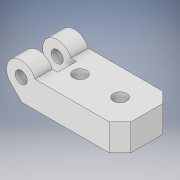
# Autodesk Inventor part: Piston Wall Guide
Saved by Autodesk Inventor 2018 (Build 220112000, 112)
## iProperties
Created: 2017-09-27
Part Number: Piston Wall Guide
Material: ASA Plastic
Document SubType Name: Modeling
Designer: Gabriel Smolnycki
Density: 1.07 g/cm^3
Appearance: Smooth - White ASA
Author: Gabriel Smolnycki
Autodesk Inventor part; units mm, degrees
ref_plane "YZ Plane" through (0, 0, 0) normal (1, 0, 0) x (0, 1, 0)
ref_plane "XZ Plane" through (0, 0, 0) normal (0, 1, 0) x (-1, 0, 0)
ref_plane "XY Plane" through (0, 0, 0) normal (0, 0, 1) x (1, 0, 0)
sketch "Sketch1" plane through (0, 0, 0) normal (0, 1, 0) x (-1, 0, 0)
  line L0 (17.5, 10) -> (-17.5, 10)
  line L1 (-17.5, 10) -> (-17.5, -10)
  line L2 (-17.5, -10) -> (17.5, -10)
  line L3 (17.5, -10) -> (17.5, 10)
  line L4 (17.5, 10) -> (-17.5, -10) construction
  line L5 (-17.5, 10) -> (17.5, -10) construction
  point P0 (0, 0)
  dimension "d0" = 35
  dimension "d1" = 20
  constraints: 12 end point, 2 midpoint, 2 parallel, 1 horizontal, 1 perpendicular
  measures "d0" distance of L2.end L1.end
  measures "d1" distance of L1.end L0.end
extrude "Extrusion1" add sketch "Sketch1" along normal blind 10
sketch "Sketch2" plane through (0, 10, 0) normal (0, 1, 0) x (1, 0, 0)
  line L0 (-17.5, 10) -> (-17.5, -10) projected
  line L1 (17.5, -10) -> (17.5, 10) projected
  point P0 (0, 0)
  point P1 (-7.5, 0)
  point P2 (7.5, 0)
  dimension "d4" = 10
  dimension "d5" = 10
  constraints: 2 horizontal alignment
  measures "d4" distance from line of point (-7.5, 0) L0
  measures "d5" distance from line of L1 point (7.5, 0)
hole "Hole1" at (-7.5, 10, 0) at (7.5, 10, 0) direction (0, -1, 0) diameter 5 end through all
sketch "Sketch3" plane through (-17.5, 0, 10) normal (0, 0, 1) x (1, 0, 0)
  arc A0 (3.1235, 10) -> (-5.8891, 4.1109) centre (-2, 8) ccw
  line L0 (0, 0) -> (0, 10) projected
  line L1 (0, 0) -> (35, 0) projected
  line L2 (-5.8891, 4.1109) -> (-1.7782, 0)
  line L3 (0, 0) -> (-1.7782, 0)
  line L4 (0, 10) -> (35, 10) projected
  point P0 (17.5, 0)
  dimension "d13" = 11
  dimension "d14" = 2
  dimension "d15" = 8
  dimension "d18" = 135
  constraints: 4 end point, 2 point on circle, 1 centre point, 1 horizontal, 1 point on line, 1 tangent
  measures "d13" diameter of A0
  measures "d14" distance from line of L0 A0.centre
  measures "d15" distance from line of L1 A0.centre
  measures "d18" angle of L3 L2
extrude "Extrusion2" add sketch "Sketch3" against normal blind 6.5
mirror "Mirror1" about plane through (0, 0, 0) normal (0, 0, 1) of "Extrusion2"
sketch "Sketch4" plane through (-17.5, 0, 3.5) normal (0, 0, -1) x (-1, 0, 0)
  arc A0 (5.8891, 4.1109) -> (-3.1235, 10) centre (2, 8) ccw projected
  circle A1 centre (2, 8) radius 7.5
  point P0 (-17.5, 0)
  dimension "d21" = 15
  constraints: 1 centre point, 1 coincident
  measures "d21" diameter of A1
extrude "Extrusion3" cut sketch "Sketch4" along normal up to surface (7 mm away)
sketch "Sketch5" plane through (17.5, 0, 10) normal (0, 0, 1) x (1, 0, 0)
  arc A0 (-31.8765, 10) -> (-40.8891, 4.1109) centre (-37, 8) ccw projected
  point P0 (-17.5, 0)
  constraints: 1 coincident
hole "Hole2" at (-19.5, 8, 10) direction (0, 0, -1) diameter 4.5 end through all
chamfer "Chamfer1" distance 4 angle 45 2 edges at (17.5, 5, 10) (17.5, 5, -10)
body "Solid1"
